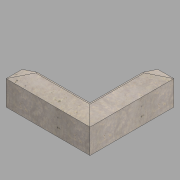
# Autodesk Inventor part: Corner_cap_5
Saved by Autodesk Inventor 2022.1 (Build 261234020, 234B)
## iProperties
Created: 2021-12-03
Part Number: Corner_cap_5
Material: Limestone
Document SubType Name: Modeling
Designer: awelt
Density: 2.6 g/cm^3
Appearance: Kasota Gray
Mass: 186744 g
Surface Area: 14696.4 cm^2
Volume: 71824.5 cm^3
Author: awelt
Autodesk Inventor part; units mm, degrees
ref_plane "YZ Plane" through (0, 0, 0) normal (1, 0, 0) x (0, 1, 0)
ref_plane "XZ Plane" through (0, 0, 0) normal (0, 1, 0) x (-1, 0, 0)
ref_plane "XY Plane" through (0, 0, 0) normal (0, 0, 1) x (1, 0, 0)
sketch "Sketch1" plane through (0, 0, 0) normal (0, 1, 0) x (-1, 0, 0)
  line L0 (0, 0) -> (698.5, 0)
  line L1 (0, 0) -> (0, -698.5)
  line L2 (0, -698.5) -> (-165.1, -698.5)
  line L3 (698.5, 0) -> (698.5, 165.1)
  line L4 (-165.1, -698.5) -> (-165.1, 165.1)
  line L5 (-165.1, 165.1) -> (698.5, 165.1)
  dimension "d1" = 698.5
  dimension "d2" = 698.5
  dimension "d3" = 165.1
  dimension "d4" = 165.1
  dimension "d5" = 863.6
  dimension "d6" = 863.6
  constraints: 12 end point, 3 vertical, 2 horizontal, 1 perpendicular
  measures "d1" distance of L0.start L0.end
  measures "d2" distance of L0.start L1.end
  measures "d3" distance of L1.end L2.end
  measures "d4" distance of L0.end L3.end
  measures "d5" distance of L2.end L4.end
  measures "d6" distance of L4.end L3.end
extrude "Extrusion1" add sketch "Sketch1" along normal blind 304.8
sketch "Sketch2" plane through (-698.5, 0, 0) normal (-1, 0, 0) x (0, 0, 1)
  line L0 (0, 304.8) -> (165.1, 304.8) projected
  line L1 (165.1, 0) -> (165.1, 304.8) projected
  line L2 (12.7, 304.8) -> (165.1, 254)
  line L3 (165.1, 254) -> (165.1, 304.8)
  line L4 (165.1, 304.8) -> (12.7, 304.8)
  point P0 (0, 0)
  dimension "d9" = 12.7
  dimension "d10" = 50.8
  constraints: 6 end point, 2 point on line, 1 collinear, 1 vertical
  measures "d9" distance of L2.start L0.start
  measures "d10" distance of L2.end L0.end
sketch3d "3D Sketch1"
  line L0 (-698.5, 304.8, 0) -> (0, 304.8, 0)
  line L1 (0, 304.8, 0) -> (0, 304.8, -698.5)
sweep "Sweep1" cut profiles "Sketch2" path "3D Sketch1"
sketch "Sketch3" plane through (0, 0, 0) normal (0, 0, -1) x (-1, 0, 0)
  line L0 (698.5, 304.8) -> (-12.7, 304.8) projected
  line L1 (698.5, 254) -> (698.5, 304.8) projected
  line L2 (698.5, 0) -> (698.5, 254) projected
  line L3 (546.1, 304.8) -> (698.5, 254)
  line L4 (698.5, 254) -> (698.5, 304.8)
  line L5 (698.5, 304.8) -> (546.1, 304.8)
  point P0 (0, 0)
  dimension "d13" = 152.4
  dimension "d14" = 50.8
  constraints: 6 end point, 2 collinear, 2 point on line
  measures "d13" distance of L3.start L0.start
  measures "d14" distance of point (698.5, 254) L0.start
extrude "Extrusion2" cut sketch "Sketch3" against normal through all
sketch "Sketch4" plane through (0, 0, -698.5) normal (-1, 0, 0) x (0, 0, 1)
  line L0 (0, 304.8) -> (698.5, 304.8) projected
  line L1 (0, 304.8) -> (0, 254) projected
  line L2 (0, 254) -> (152.4, 304.8)
  line L3 (152.4, 304.8) -> (0, 304.8)
  line L4 (0, 304.8) -> (0, 254)
  point P0 (698.5, 0)
  point P1 (0, 254)
  dimension "d17" = 152.4
  dimension "d18" = 50.8
  constraints: 6 end point, 2 collinear, 2 point on line
  measures "d17" distance of L2.end L0.start
  measures "d18" distance of point (0, 254) L0.start
extrude "Extrusion3" cut sketch "Sketch4" against normal through all
equation "\"d2\" = d1"
equation "\"d4\" = d3"
body "Solid1"
